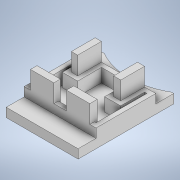
# Autodesk Inventor part: FlanecForwardBabka
Saved by Autodesk Inventor 2022 (Build 260153000, 153)
## iProperties
Created: 2023-08-16
Part Number: FlanecForwardBabka
Material: Generic
Document SubType Name: Modeling
Designer: Kippi
Density: 1 g/cm^3
Appearance: Default
Author: Kippi
Autodesk Inventor part; units mm, degrees
ref_plane "YZ Plane" through (0, 0, 0) normal (1, 0, 0) x (0, 1, 0)
ref_plane "XZ Plane" through (0, 0, 0) normal (0, 1, 0) x (-1, 0, 0)
ref_plane "XY Plane" through (0, 0, 0) normal (0, 0, 1) x (1, 0, 0)
sketch "Sketch1" plane through (0, 0, 0) normal (0, 1, 0) x (-1, 0, 0)
  line L0 (49.875, 66.5) -> (-110.125, 66.5)
  line L1 (-110.125, 66.5) -> (-110.125, -66.5)
  line L2 (-110.125, -66.5) -> (49.875, -66.5)
  line L3 (49.875, -66.5) -> (49.875, 66.5)
  line L4 (24.875, -66.5) -> (-85.125, -66.5)
  line L5 (-85.125, -66.5) -> (-85.125, -219)
  line L6 (-85.125, -219) -> (24.875, -219)
  line L7 (24.875, -219) -> (24.875, -66.5)
  point P0 (0, 0)
  dimension "d0" = 133
  dimension "d1" = 160
  dimension "d2" = 25
  dimension "d3" = 25
  dimension "d4" = 110
  constraints: 16 end point, 4 parallel, 2 horizontal, 2 perpendicular, 1 point on line
  measures "d0" distance of L2.end L0.start
  measures "d1" distance of L1.end L2.end
  measures "d2" distance between parallel lines of L1 L5
  measures "d3" distance between parallel lines of L3 L7
  measures "d4" distance of L5.end L6.end
extrude "Extrusion1" add sketch "Sketch1" along normal blind 40 contours L3 L2 L1 L0
sketch "Sketch2" plane through (0, 40, 0) normal (0, 1, 0) x (1, 0, 0)
  line L0 (110.125, 66.5) -> (-49.875, 66.5) construction
  line L1 (-49.875, 66.5) -> (-49.875, -66.5) construction
  line L2 (-49.875, -66.5) -> (110.125, -66.5) construction
  line L3 (110.125, -66.5) -> (110.125, 66.5) construction
  line L4 (-24.875, 66.5) -> (-10.8349, 66.5)
  line L5 (-10.8349, 66.5) -> (-10.8349, 13.5)
  line L6 (-10.8349, 13.5) -> (-24.875, 13.5)
  line L7 (-24.875, 13.5) -> (-24.875, 66.5)
  line L8 (85.125, 66.5) -> (69.2723, 66.5)
  line L9 (69.2723, 66.5) -> (69.2723, 13.5)
  line L10 (69.2723, 13.5) -> (85.125, 13.5)
  line L11 (85.125, 13.5) -> (85.125, 66.5)
  point P0 (0, 0)
  dimension "d7" = 25
  dimension "d8" = 25
  dimension "d11" = 80
  dimension "d12" = 80
  dimension "d13" = 110
  constraints: 16 end point, 4 parallel, 2 horizontal, 2 perpendicular, 2 point on line
  measures "d7" distance between parallel lines of L3 L11
  measures "d8" distance between parallel lines of L1 L7
  measures "d11" distance between parallel lines of L2 L10
  measures "d12" distance between parallel lines of L6 L2
  measures "d13" distance between parallel lines of L11 L7
extrude "Extrusion2" add sketch "Sketch2" along normal blind 40
sketch "Sketch3" plane through (0, 40, 0) normal (0, 1, 0) x (1, 0, 0)
  line L0 (85.125, 66.5) -> (85.125, 13.5) construction
  line L1 (85.125, 13.5) -> (69.2723, 13.5) construction
  line L2 (69.2723, 13.5) -> (69.2723, 66.5) construction
  line L3 (69.2723, 66.5) -> (-10.8349, 66.5) construction
  line L4 (-10.8349, 66.5) -> (-10.8349, 13.5) construction
  line L5 (-10.8349, 13.5) -> (-24.875, 13.5) construction
  line L6 (-24.875, 13.5) -> (-24.875, 66.5) construction
  line L7 (-24.875, 66.5) -> (-49.875, 66.5) construction
  line L8 (-49.875, 66.5) -> (-49.875, -66.5) construction
  line L9 (-49.875, -66.5) -> (110.125, -66.5) construction
  line L10 (110.125, -66.5) -> (110.125, 66.5) construction
  line L11 (110.125, 66.5) -> (85.125, 66.5) construction
  line L12 (-39.875, -56.5) -> (-39.875, 56.5)
  line L13 (-39.875, 56.5) -> (-34.875, 56.5)
  line L14 (-34.875, 56.5) -> (-34.875, 3.5)
  line L15 (-34.875, 3.5) -> (-0.8349, 3.5)
  line L16 (-0.8349, 3.5) -> (-0.8349, 56.5)
  line L17 (-0.8349, 56.5) -> (59.2723, 56.5)
  line L18 (59.2723, 56.5) -> (59.2723, 3.5)
  line L19 (59.2723, 3.5) -> (95.125, 3.5)
  line L20 (95.125, 3.5) -> (95.125, 56.5)
  line L21 (95.125, 56.5) -> (100.125, 56.5)
  line L22 (100.125, 56.5) -> (100.125, -56.5)
  line L23 (100.125, -56.5) -> (-39.875, -56.5)
  point P0 (0, 0)
  dimension "d16" = 10
  constraints: 24 end point, 11 other
  measures "d16" distance between parallel lines of L8 L12
extrude "Extrusion3" cut sketch "Sketch3" against normal blind 30
sketch "Sketch4" plane through (0, 40, 0) normal (0, 1, 0) x (1, 0, 0)
  line L0 (-49.875, 66.5) -> (-49.875, -66.5) construction
  line L1 (-49.875, -66.5) -> (110.125, -66.5) construction
  line L2 (110.125, -66.5) -> (110.125, 66.5) construction
  line L3 (-35.875, -66.5) -> (16.125, -66.5)
  line L4 (16.125, -66.5) -> (16.125, -52)
  line L5 (16.125, -52) -> (-35.875, -52)
  line L6 (-35.875, -52) -> (-35.875, -66.5)
  line L7 (96.125, -66.5) -> (44.125, -66.5)
  line L8 (44.125, -66.5) -> (44.125, -50)
  line L9 (44.125, -50) -> (96.125, -50)
  line L10 (96.125, -50) -> (96.125, -66.5)
  point P0 (0, 0)
  dimension "d19" = 28
  dimension "d20" = 14
  dimension "d21" = 14
  dimension "d24" = 52
  dimension "d25" = 52
  constraints: 16 end point, 4 parallel, 2 horizontal, 2 perpendicular, 2 point on line
  measures "d19" distance between parallel lines of L4 L8
  measures "d20" distance between parallel lines of L2 L10
  measures "d21" distance between parallel lines of L0 L6
  measures "d24" distance of L4.end L5.end
  measures "d25" distance of L8.end L9.end
extrude "Extrusion4" add sketch "Sketch4" along normal mid plane 80
sketch "Sketch5" plane through (110.125, 0, 66.5) normal (1, 0, 0) x (0, 0, -1)
  line L0 (133, 0) -> (133, 40) construction
  line L1 (133, 0) -> (173, 0)
  line L2 (173, 0) -> (173, 20)
  line L3 (173, 20) -> (133, 20)
  line L4 (133, 20) -> (133, 0)
  line L5 (0, 0) -> (-40, 0)
  line L6 (-40, 0) -> (-40, 20)
  line L7 (-40, 20) -> (0, 20)
  line L8 (0, 20) -> (0, 0)
  point P0 (66.5, 0)
  dimension "d26" = 20
  dimension "d27" = 40
  dimension "d30" = 40
  constraints: 16 end point, 4 parallel, 2 horizontal, 2 perpendicular
  measures "d26" distance between parallel lines of L1 L3
  measures "d27" distance between parallel lines of L0 L2
  measures "d30" distance of L6.end L7.end
extrude "Extrusion5" add sketch "Sketch5" against normal up to surface (160 mm away)
sketch "Sketch6" plane through (0, 0, 0) normal (0, -1, 0) x (1, 0, 0)
  line L0 (110.125, -106.5) -> (-49.875, -106.5) construction
  circle A0 centre (30.125, -236.5) radius 150
  point P0 (0, 0)
  dimension "d31" = 130
  dimension "d32" = 300
  constraints: 1 centre point
  measures "d31" distance from line of L0 A0.centre
  measures "d32" diameter of A0
extrude "Extrusion6" cut sketch "Sketch6" against normal blind 100
body "Solid1"
